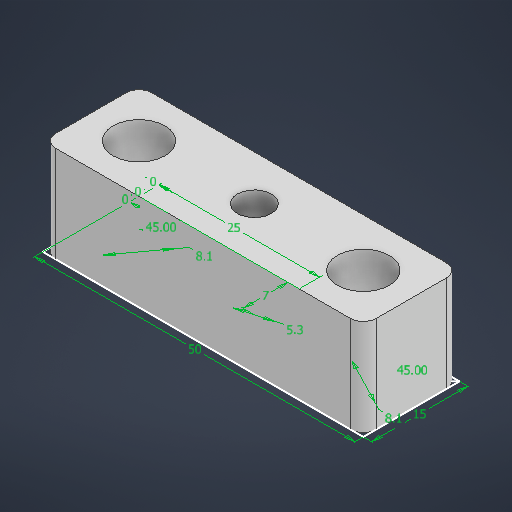
# Autodesk Inventor part: Support_Seperator(Middle rod)
Saved by Autodesk Inventor 2026.2 (Build 302298000, 298)
## iProperties
Created: 2025-12-17
Part Number: Support_Seperator(Middle rod)
Material: Generic
Document SubType Name: Modeling
Designer: Cobble
Density: 1 g/cm^3
Appearance: Default
Author: Cobble
Autodesk Inventor part; units mm, degrees
ref_plane "YZ Plane" through (0, 0, 0) normal (1, 0, 0) x (0, 1, 0)
ref_plane "XZ Plane" through (0, 0, 0) normal (0, 1, 0) x (-1, 0, 0)
ref_plane "XY Plane" through (0, 0, 0) normal (0, 0, 1) x (1, 0, 0)
sketch "Sketch1" plane through (0, 0, 0) normal (0, 0, 1) x (1, 0, 0)
  line L0 (0, 0) -> (50, 0)
  line L1 (50, 0) -> (50, -15)
  line L2 (50, -15) -> (0, -15)
  line L3 (0, -15) -> (0, 0)
  line L4 (0, 0) -> (15, -15)
  line L5 (0, 0) -> (21.2132, 0) construction
  circle A0 centre (7.5, -7.5) radius 4.05
  line L6 (50, 0) -> (35, -15)
  circle A1 centre (42.5, -7.5) radius 4.05
  circle A2 centre (25, -7) radius 2.65
  circle A3 centre (7.5, -7.5) radius 7.5
  circle A4 centre (42.5, -7.5) radius 7.5
  line L7 (25, -7) -> (25, 0)
  point P0 (0, 0)
  dimension "d0" = 50
  dimension "d1" = 15
  dimension "d2" = 45
  dimension "d3" = 8.1
  dimension "d4" = 8.1
  dimension "d5" = 45
  dimension "d9" = 0
  dimension "d13" = 0
  dimension "d14" = 5.3
  dimension "d18" = 7
  dimension "d19" = 25
  dimension "d20" = 0
  constraints: 16 end point, 5 centre point, 2 coincident, 2 horizontal, 2 midpoint, 2 parallel, 2 perpendicular, 2 point on line, 2 tangent, 1 equal length, 1 vertical
  measures "d0" distance of L2.start L2.end
  measures "d1" distance of L0.end L2.start
  measures "d2" angle of L4 L5
  measures "d3" diameter of A0
  measures "d4" diameter of A1
  measures "d5" angle of L0 L6
  measures "d9" horizontal distance of point (0, 0) L2.end
  measures "d13" distance of point (0, 0) L0.start
  measures "d14" diameter of A2
  measures "d18" distance of L7.start L7.end
  measures "d19" distance of point (0, 0) L7.end
  measures "d20" vertical distance of point (0, 0) L7.end
extrude "Extrusion1" add sketch "Sketch1" along normal blind 15 contours L4 A3 L3 | L0 A3 L4 | L0 A4 L6 L2 L4 A3 | A3 L4 A0 | A3 L2 L3 | A3 L4 A0 | A3 L4 L2 | L0 L6 A4 | A4 L6 A1 | L1 A4 L6 | A4 L6 A1 | A4 L2 L6 | L1 L2 A4
fillet "Fillet1" radius 2 4 edges at (50, -15, 7.5) (50, 0, 7.5) (0, -15, 7.5) (0, 0, 7.5)
body "Solid1"
